Autodesk Fusion 360 part; units mm, degrees
note: some values were not read from the file. Set by a fixed rule: which sketch regions a step uses.
(part 19 of 59)
  spline S107 degree 5 poles (23.3609, -7.8781) (23.3596, -7.8757) (23.3571, -7.871) (23.3532, -7.8639) (23.348, -7.8544) (23.3416, -7.8426) (23.3351, -7.8308) (23.3287, -7.819) (23.3222, -7.8073) (23.3158, -7.7957) (23.3094, -7.784) (23.3029, -7.7724) (23.2965, -7.7609) (23.29, -7.7493) (23.2836, -7.7379) (23.2771, -7.7264) (23.2707, -7.715) (23.2643, -7.7036) (23.2578, -7.6922) (23.2514, -7.6809) (23.245, -7.6697) (23.2385, -7.6584) (23.2321, -7.6472) (23.2257, -7.636) (23.2193, -7.6249) (23.2128, -7.6138) (23.2064, -7.6028) (23.2, -7.5917) (23.1936, -7.5808) (23.1872, -7.5698) (23.1807, -7.5589) (23.1743, -7.548) (23.1679, -7.5372) (23.1615, -7.5264) (23.1551, -7.5156) (23.1487, -7.5049) (23.1423, -7.4942) (23.136, -7.4836) (23.1296, -7.473) (23.1232, -7.4624) (23.1168, -7.4518) (23.1104, -7.4413) (23.1041, -7.4309) (23.0977, -7.4205) (23.0914, -7.4101) (23.085, -7.3997) (23.0786, -7.3894) (23.0723, -7.3791) (23.066, -7.3689) (23.0596, -7.3587) (23.0533, -7.3486) (23.047, -7.3384) (23.0406, -7.3284) (23.0343, -7.3183) (23.028, -7.3083) (23.0217, -7.2984) (23.0154, -7.2884) (23.0091, -7.2785) (23.0029, -7.2687) (22.9966, -7.2589) (22.9903, -7.2491) (22.984, -7.2394) (22.9778, -7.2297) (22.9715, -7.22) (22.9653, -7.2104) (22.9591, -7.2009) (22.9528, -7.1913) (22.9466, -7.1818) (22.9404, -7.1724) (22.9342, -7.163) (22.928, -7.1536) (22.9218, -7.1443) (22.9156, -7.135) (22.9095, -7.1257) (22.9033, -7.1165) (22.8971, -7.1073) (22.891, -7.0982) (22.8849, -7.0891) (22.8787, -7.0801) (22.8726, -7.0711) (22.8665, -7.0621) (22.8604, -7.0532) (22.8543, -7.0443) (22.8483, -7.0354) (22.8422, -7.0266) (22.8361, -7.0179) (22.8301, -7.0091) (22.8241, -7.0005) (22.818, -6.9918) (22.812, -6.9832) (22.806, -6.9747) (22.8, -6.9662) (22.7941, -6.9577) (22.7881, -6.9493) (22.7822, -6.9409) (22.7762, -6.9325) (22.7703, -6.9242) (22.7644, -6.916) (22.7585, -6.9078) (22.7526, -6.8996) (22.7467, -6.8914) (22.7408, -6.8834) (22.735, -6.8753) (22.7292, -6.8673) (22.7233, -6.8593) (22.7175, -6.8514) (22.7118, -6.8436) (22.706, -6.8357) (22.7002, -6.8279) (22.6945, -6.8202) (22.6887, -6.8125) (22.683, -6.8048) (22.6773, -6.7972) (22.6716, -6.7897) (22.666, -6.7821) (22.6603, -6.7747) (22.6547, -6.7672) (22.6491, -6.7598) (22.6435, -6.7525) (22.6379, -6.7452) (22.6323, -6.7379) (22.6268, -6.7307) (22.6212, -6.7236) (22.6157, -6.7165) (22.6102, -6.7094) (22.6048, -6.7024) (22.5993, -6.6954) (22.5939, -6.6884) (22.5884, -6.6815) (22.583, -6.6747) (22.5777, -6.6679) (22.5723, -6.6611) (22.567, -6.6544) (22.5617, -6.6478) (22.5564, -6.6412) (22.5511, -6.6346) (22.5458, -6.6281) (22.5406, -6.6216) (22.5354, -6.6152) (22.5302, -6.6088) (22.525, -6.6025) (22.5199, -6.5962) (22.5148, -6.59) (22.5097, -6.5838) (22.5046, -6.5776) (22.4996, -6.5715) (22.4945, -6.5655) (22.4895, -6.5595) (22.4846, -6.5536) (22.4796, -6.5477) (22.4747, -6.5418) (22.4698, -6.536) (22.4649, -6.5303) (22.4601, -6.5246) (22.4553, -6.5189) (22.4505, -6.5133) (22.4457, -6.5077) (22.441, -6.5022) (22.4363, -6.4968) (22.4316, -6.4914) (22.427, -6.486) (22.4223, -6.4807) (22.4177, -6.4755) (22.4132, -6.4703) (22.4087, -6.4651) (22.4042, -6.46) (22.3997, -6.455) (22.3953, -6.45) (22.3909, -6.4451) (22.3865, -6.4402) (22.3821, -6.4353) (22.3778, -6.4306) (22.3736, -6.4258) (22.3693, -6.4211) (22.3651, -6.4165) (22.3609, -6.4119) (22.3568, -6.4074) (22.3527, -6.403) (22.3486, -6.3986) (22.3446, -6.3942) (22.3406, -6.3899) (22.3367, -6.3856) (22.3328, -6.3814) (22.3289, -6.3773) (22.325, -6.3732) (22.3212, -6.3692) (22.3175, -6.3652) (22.3138, -6.3613) (22.3101, -6.3574) (22.3065, -6.3536) (22.3029, -6.3499) (22.2993, -6.3462) (22.2958, -6.3426) (22.2923, -6.339) (22.2889, -6.3355) (22.2855, -6.332) (22.2822, -6.3286) (22.2789, -6.3252) (22.2757, -6.322) (22.2725, -6.3187) (22.2693, -6.3156) (22.2662, -6.3124) (22.2632, -6.3094) (22.2602, -6.3064) (22.2572, -6.3035) (22.2543, -6.3006) (22.2515, -6.2978) (22.2487, -6.2951) (22.2459, -6.2924) (22.2433, -6.2897) (22.2406, -6.2872) (22.238, -6.2847) (22.2355, -6.2823) (22.2331, -6.2799) (22.2307, -6.2776) (22.2283, -6.2753) (22.226, -6.2732) (22.2238, -6.271) (22.2216, -6.269) (22.2195, -6.267) (22.2175, -6.2651) (22.2155, -6.2632) (22.2136, -6.2615) (22.2117, -6.2597) (22.2099, -6.2581) (22.2082, -6.2565) (22.2066, -6.255) (22.205, -6.2536) (22.2035, -6.2522) (22.202, -6.2509) (22.2007, -6.2497) (22.1994, -6.2485) (22.1982, -6.2474) (22.197, -6.2464) (22.196, -6.2455) (22.195, -6.2446) (22.1941, -6.2438) (22.1933, -6.2431) (22.1925, -6.2424) (22.1919, -6.2419) (22.1913, -6.2414) (22.1909, -6.241) (22.1907, -6.2408) (22.1905, -6.2407) (22.1904, -6.2406) knots -1 -1 -1 -1 -1 -1 -0.99583333 -0.99166667 -0.9875 -0.98333333 -0.97916667 -0.975 -0.97083333 -0.96666667 -0.9625 -0.95833333 -0.95416667 -0.95 -0.94583333 -0.94166667 -0.9375 -0.93333333 -0.92916667 -0.925 -0.92083333 -0.91666667 -0.9125 -0.90833333 -0.90416667 -0.9 -0.89583333 -0.89166667 -0.8875 -0.88333333 -0.87916667 -0.875 -0.87083333 -0.86666667 -0.8625 -0.85833333 -0.85416667 -0.85 -0.84583333 -0.84166667 -0.8375 -0.83333333 -0.82916667 -0.825 -0.82083333 -0.81666667 -0.8125 -0.80833333 -0.80416667 -0.8 -0.79583333 -0.79166667 -0.7875 -0.78333333 -0.77916667 -0.775 -0.77083333 -0.76666667 -0.7625 -0.75833333 -0.75416667 -0.75 -0.74583333 -0.74166667 -0.7375 -0.73333333 -0.72916667 -0.725 -0.72083333 -0.71666667 -0.7125 -0.70833333 -0.70416667 -0.7 -0.69583333 -0.69166667 -0.6875 -0.68333333 -0.67916667 -0.675 -0.67083333 -0.66666667 -0.6625 -0.65833333 -0.65416667 -0.65 -0.64583333 -0.64166667 -0.6375 -0.63333333 -0.62916667 -0.625 -0.62083333 -0.61666667 -0.6125 -0.60833333 -0.60416667 -0.6 -0.59583333 -0.59166667 -0.5875 -0.58333333 -0.57916667 -0.575 -0.57083333 -0.56666667 -0.5625 -0.55833333 -0.55416667 -0.55 -0.54583333 -0.54166667 -0.5375 -0.53333333 -0.52916667 -0.525 -0.52083333 -0.51666667 -0.5125 -0.50833333 -0.50416667 -0.5 -0.49583333 -0.49166667 -0.4875 -0.48333333 -0.47916667 -0.475 -0.47083333 -0.46666667 -0.4625 -0.45833333 -0.45416667 -0.45 -0.44583333 -0.44166667 -0.4375 -0.43333333 -0.42916667 -0.425 -0.42083333 -0.41666667 -0.4125 -0.40833333 -0.40416667 -0.4 -0.39583333 -0.39166667 -0.3875 -0.38333333 -0.37916667 -0.375 -0.37083333 -0.36666667 -0.3625 -0.35833333 -0.35416667 -0.35 -0.34583333 -0.34166667 -0.3375 -0.33333333 -0.32916667 -0.325 -0.32083333 -0.31666667 -0.3125 -0.30833333 -0.30416667 -0.3 -0.29583333 -0.29166667 -0.2875 -0.28333333 -0.27916667 -0.275 -0.27083333 -0.26666667 -0.2625 -0.25833333 -0.25416667 -0.25 -0.24583333 -0.24166667 -0.2375 -0.23333333 -0.22916667 -0.225 -0.22083333 -0.21666667 -0.2125 -0.20833333 -0.20416667 -0.2 -0.19583333 -0.19166667 -0.1875 -0.18333333 -0.17916667 -0.175 -0.17083333 -0.16666667 -0.1625 -0.15833333 -0.15416667 -0.15 -0.14583333 -0.14166667 -0.1375 -0.13333333 -0.12916667 -0.125 -0.12083333 -0.11666667 -0.1125 -0.10833333 -0.10416667 -0.1 -0.09583333 -0.09166667 -0.0875 -0.08333333 -0.07916667 -0.075 -0.07083333 -0.06666667 -0.0625 -0.05833333 -0.05416667 -0.05 -0.04583333 -0.04166667 -0.0375 -0.03333333 -0.02916667 -0.025 -0.02083333 -0.01666667 -0.0125 -0.00833333 -0.00416667 0 0 0 0 0 0
  spline S108 degree 5 poles (-30.2174, 5.5786) (-30.2148, 5.5782) (-30.2094, 5.5775) (-30.2014, 5.5764) (-30.1907, 5.575) (-30.1773, 5.5733) (-30.164, 5.5716) (-30.1507, 5.5699) (-30.1375, 5.5683) (-30.1242, 5.5666) (-30.111, 5.565) (-30.0979, 5.5634) (-30.0847, 5.5618) (-30.0716, 5.5602) (-30.0585, 5.5587) (-30.0455, 5.5572) (-30.0324, 5.5557) (-30.0194, 5.5542) (-30.0065, 5.5527) (-29.9935, 5.5513) (-29.9806, 5.5499) (-29.9678, 5.5484) (-29.9549, 5.5471) (-29.9421, 5.5457) (-29.9293, 5.5444) (-29.9166, 5.543) (-29.9039, 5.5417) (-29.8912, 5.5404) (-29.8785, 5.5392) (-29.8659, 5.5379) (-29.8533, 5.5367) (-29.8407, 5.5355) (-29.8282, 5.5343) (-29.8157, 5.5331) (-29.8032, 5.532) (-29.7908, 5.5309) (-29.7784, 5.5298) (-29.766, 5.5287) (-29.7537, 5.5276) (-29.7414, 5.5265) (-29.7291, 5.5255) (-29.7169, 5.5245) (-29.7047, 5.5235) (-29.6925, 5.5225) (-29.6803, 5.5216) (-29.6682, 5.5206) (-29.6562, 5.5197) (-29.6441, 5.5188) (-29.6321, 5.5179) (-29.6201, 5.517) (-29.6082, 5.5162) (-29.5963, 5.5154) (-29.5844, 5.5145) (-29.5726, 5.5137) (-29.5608, 5.513) (-29.549, 5.5122) (-29.5373, 5.5115) (-29.5256, 5.5108) (-29.514, 5.51) (-29.5023, 5.5094) (-29.4907, 5.5087) (-29.4792, 5.508) (-29.4677, 5.5074) (-29.4562, 5.5068) (-29.4447, 5.5062) (-29.4333, 5.5056) (-29.422, 5.505) (-29.4106, 5.5045) (-29.3993, 5.504) (-29.3881, 5.5035) (-29.3768, 5.503) (-29.3657, 5.5025) (-29.3545, 5.502) (-29.3434, 5.5016) (-29.3323, 5.5011) (-29.3213, 5.5007) (-29.3103, 5.5003) (-29.2993, 5.4999) (-29.2884, 5.4996) (-29.2775, 5.4992) (-29.2667, 5.4989) (-29.2559, 5.4986) (-29.2451, 5.4983) (-29.2344, 5.498) (-29.2237, 5.4977) (-29.213, 5.4975) (-29.2024, 5.4972) (-29.1919, 5.497) (-29.1813, 5.4968) (-29.1708, 5.4966) (-29.1604, 5.4965) (-29.15, 5.4963) (-29.1396, 5.4962) (-29.1293, 5.496) (-29.119, 5.4959) (-29.1088, 5.4958) (-29.0986, 5.4957) (-29.0884, 5.4957) (-29.0783, 5.4956) (-29.0682, 5.4956) (-29.0582, 5.4955) (-29.0482, 5.4955) (-29.0383, 5.4955) (-29.0284, 5.4955) (-29.0185, 5.4956) (-29.0087, 5.4956) (-28.9989, 5.4957) (-28.9892, 5.4957) (-28.9795, 5.4958) (-28.9698, 5.4959) (-28.9602, 5.496) (-28.9507, 5.4962) (-28.9412, 5.4963) (-28.9317, 5.4964) (-28.9223, 5.4966) (-28.9129, 5.4968) (-28.9036, 5.497) (-28.8943, 5.4972) (-28.8851, 5.4974) (-28.8759, 5.4976) (-28.8668, 5.4979) (-28.8577, 5.4981) (-28.8486, 5.4984) (-28.8396, 5.4986) (-28.8307, 5.4989) (-28.8218, 5.4992) (-28.8129, 5.4995) (-28.8041, 5.4999) (-28.7953, 5.5002) (-28.7866, 5.5005) (-28.778, 5.5009) (-28.7694, 5.5013) (-28.7608, 5.5016) (-28.7523, 5.502) (-28.7438, 5.5024) (-28.7354, 5.5028) (-28.727, 5.5032) (-28.7187, 5.5037) (-28.7105, 5.5041) (-28.7023, 5.5046) (-28.6941, 5.505) (-28.686, 5.5055) (-28.678, 5.506) (-28.67, 5.5064) (-28.662, 5.5069) (-28.6541, 5.5074) (-28.6463, 5.5079) (-28.6385, 5.5085) (-28.6307, 5.509) (-28.6231, 5.5095) (-28.6154, 5.5101) (-28.6079, 5.5106) (-28.6004, 5.5112) (-28.5929, 5.5118) (-28.5855, 5.5123) (-28.5781, 5.5129) (-28.5709, 5.5135) (-28.5636, 5.5141) (-28.5564, 5.5147) (-28.5493, 5.5153) (-28.5423, 5.5159) (-28.5353, 5.5165) (-28.5283, 5.5172) (-28.5214, 5.5178) (-28.5146, 5.5184) (-28.5078, 5.5191) (-28.5011, 5.5197) (-28.4945, 5.5204) (-28.4879, 5.5211) (-28.4814, 5.5217) (-28.4749, 5.5224) (-28.4685, 5.5231) (-28.4622, 5.5237) (-28.4559, 5.5244) (-28.4497, 5.5251) (-28.4435, 5.5258) (-28.4374, 5.5265) (-28.4314, 5.5272) (-28.4255, 5.5279) (-28.4196, 5.5286) (-28.4137, 5.5293) (-28.408, 5.53) (-28.4023, 5.5307) (-28.3966, 5.5314) (-28.3911, 5.5321) (-28.3856, 5.5328) (-28.3802, 5.5335) (-28.3748, 5.5342) (-28.3695, 5.5349) (-28.3643, 5.5356) (-28.3592, 5.5363) (-28.3541, 5.537) (-28.3491, 5.5377) (-28.3442, 5.5384) (-28.3393, 5.5391) (-28.3345, 5.5398) (-28.3298, 5.5405) (-28.3252, 5.5412) (-28.3206, 5.5419) (-28.3161, 5.5426) (-28.3117, 5.5432) (-28.3074, 5.5439) (-28.3031, 5.5446) (-28.2989, 5.5453) (-28.2948, 5.5459) (-28.2908, 5.5466) (-28.2868, 5.5472) (-28.283, 5.5479) (-28.2792, 5.5485) (-28.2755, 5.5492) (-28.2719, 5.5498) (-28.2683, 5.5504) (-28.2649, 5.551) (-28.2615, 5.5516) (-28.2582, 5.5522) (-28.255, 5.5528) (-28.2519, 5.5534) (-28.2489, 5.5539) (-28.246, 5.5545) (-28.2431, 5.555) (-28.2404, 5.5555) (-28.2377, 5.5561) (-28.2351, 5.5566) (-28.2327, 5.5571) (-28.2303, 5.5575) (-28.228, 5.558) (-28.2258, 5.5584) (-28.2237, 5.5589) (-28.2217, 5.5593) (-28.2198, 5.5597) (-28.218, 5.5601) (-28.2163, 5.5604) (-28.2147, 5.5608) (-28.2132, 5.5611) (-28.2118, 5.5614) (-28.2106, 5.5617) (-28.2094, 5.5619) (-28.2083, 5.5622) (-28.2074, 5.5624) (-28.2065, 5.5626) (-28.2058, 5.5628) (-28.2053, 5.5629) (-28.205, 5.563) (-28.2048, 5.563) (-28.2047, 5.563) knots -1 -1 -1 -1 -1 -1 -0.99583333 -0.99166667 -0.9875 -0.98333333 -0.97916667 -0.975 -0.97083333 -0.96666667 -0.9625 -0.95833333 -0.95416667 -0.95 -0.94583333 -0.94166667 -0.9375 -0.93333333 -0.92916667 -0.925 -0.92083333 -0.91666667 -0.9125 -0.90833333 -0.90416667 -0.9 -0.89583333 -0.89166667 -0.8875 -0.88333333 -0.87916667 -0.875 -0.87083333 -0.86666667 -0.8625 -0.85833333 -0.85416667 -0.85 -0.84583333 -0.84166667 -0.8375 -0.83333333 -0.82916667 -0.825 -0.82083333 -0.81666667 -0.8125 -0.80833333 -0.80416667 -0.8 -0.79583333 -0.79166667 -0.7875 -0.78333333 -0.77916667 -0.775 -0.77083333 -0.76666667 -0.7625 -0.75833333 -0.75416667 -0.75 -0.74583333 -0.74166667 -0.7375 -0.73333333 -0.72916667 -0.725 -0.72083333 -0.71666667 -0.7125 -0.70833333 -0.70416667 -0.7 -0.69583333 -0.69166667 -0.6875 -0.68333333 -0.67916667 -0.675 -0.67083333 -0.66666667 -0.6625 -0.65833333 -0.65416667 -0.65 -0.64583333 -0.64166667 -0.6375 -0.63333333 -0.62916667 -0.625 -0.62083333 -0.61666667 -0.6125 -0.60833333 -0.60416667 -0.6 -0.59583333 -0.59166667 -0.5875 -0.58333333 -0.57916667 -0.575 -0.57083333 -0.56666667 -0.5625 -0.55833333 -0.55416667 -0.55 -0.54583333 -0.54166667 -0.5375 -0.53333333 -0.52916667 -0.525 -0.52083333 -0.51666667 -0.5125 -0.50833333 -0.50416667 -0.5 -0.49583333 -0.49166667 -0.4875 -0.48333333 -0.47916667 -0.475 -0.47083333 -0.46666667 -0.4625 -0.45833333 -0.45416667 -0.45 -0.44583333 -0.44166667 -0.4375 -0.43333333 -0.42916667 -0.425 -0.42083333 -0.41666667 -0.4125 -0.40833333 -0.40416667 -0.4 -0.39583333 -0.39166667 -0.3875 -0.38333333 -0.37916667 -0.375 -0.37083333 -0.36666667 -0.3625 -0.35833333 -0.35416667 -0.35 -0.34583333 -0.34166667 -0.3375 -0.33333333 -0.32916667 -0.325 -0.32083333 -0.31666667 -0.3125 -0.30833333 -0.30416667 -0.3 -0.29583333 -0.29166667 -0.2875 -0.28333333 -0.27916667 -0.275 -0.27083333 -0.26666667 -0.2625 -0.25833333 -0.25416667 -0.25 -0.24583333 -0.24166667 -0.2375 -0.23333333 -0.22916667 -0.225 -0.22083333 -0.21666667 -0.2125 -0.20833333 -0.20416667 -0.2 -0.19583333 -0.19166667 -0.1875 -0.18333333 -0.17916667 -0.175 -0.17083333 -0.16666667 -0.1625 -0.15833333 -0.15416667 -0.15 -0.14583333 -0.14166667 -0.1375 -0.13333333 -0.12916667 -0.125 -0.12083333 -0.11666667 -0.1125 -0.10833333 -0.10416667 -0.1 -0.09583333 -0.09166667 -0.0875 -0.08333333 -0.07916667 -0.075 -0.07083333 -0.06666667 -0.0625 -0.05833333 -0.05416667 -0.05 -0.04583333 -0.04166667 -0.0375 -0.03333333 -0.02916667 -0.025 -0.02083333 -0.01666667 -0.0125 -0.00833333 -0.00416667 0 0 0 0 0 0
  line L236 (-26.8948, 1.5341) -> (-26.8955, 1.5338)
  spline S109 degree 5 poles (18.6136, -12.2898) (18.6128, -12.2872) (18.6113, -12.282) (18.609, -12.2743) (18.6059, -12.2639) (18.6021, -12.251) (18.5982, -12.2382) (18.5943, -12.2253) (18.5905, -12.2125) (18.5866, -12.1998) (18.5827, -12.1871) (18.5788, -12.1744) (18.5749, -12.1617) (18.571, -12.1491) (18.5671, -12.1365) (18.5632, -12.124) (18.5593, -12.1115) (18.5553, -12.099) (18.5514, -12.0866) (18.5475, -12.0742) (18.5435, -12.0618) (18.5395, -12.0495) (18.5356, -12.0372) (18.5316, -12.0249) (18.5277, -12.0127) (18.5237, -12.0005) (18.5197, -11.9884) (18.5157, -11.9762) (18.5117, -11.9642) (18.5077, -11.9521) (18.5037, -11.9401) (18.4997, -11.9281) (18.4957, -11.9162) (18.4917, -11.9043) (18.4877, -11.8925) (18.4836, -11.8806) (18.4796, -11.8689) (18.4756, -11.8571) (18.4715, -11.8454) (18.4675, -11.8337) (18.4634, -11.8221) (18.4594, -11.8105) (18.4553, -11.799) (18.4513, -11.7874) (18.4472, -11.776) (18.4431, -11.7645) (18.4391, -11.7531) (18.435, -11.7417) (18.4309, -11.7304) (18.4269, -11.7191) (18.4228, -11.7079) (18.4187, -11.6967) (18.4146, -11.6855) (18.4105, -11.6744) (18.4064, -11.6633) (18.4023, -11.6522) (18.3982, -11.6412) (18.3941, -11.6302) (18.39, -11.6193) (18.3859, -11.6084) (18.3818, -11.5975) (18.3777, -11.5867) (18.3736, -11.5759) (18.3695, -11.5652) (18.3654, -11.5545) (18.3613, -11.5438) (18.3572, -11.5332) (18.3531, -11.5226) (18.349, -11.5121) (18.3449, -11.5016) (18.3408, -11.4911) (18.3366, -11.4807) (18.3325, -11.4703) (18.3284, -11.46) (18.3243, -11.4497) (18.3202, -11.4395) (18.3161, -11.4292) (18.312, -11.4191) (18.3079, -11.409) (18.3038, -11.3989) (18.2996, -11.3888) (18.2955, -11.3788) (18.2914, -11.3689) (18.2873, -11.359) (18.2832, -11.3491) (18.2791, -11.3393) (18.275, -11.3295) (18.2709, -11.3197) (18.2668, -11.31) (18.2627, -11.3004) (18.2587, -11.2907) (18.2546, -11.2812) (18.2505, -11.2716) (18.2464, -11.2622) (18.2423, -11.2527) (18.2383, -11.2433) (18.2342, -11.234) (18.2301, -11.2247) (18.226, -11.2154) (18.222, -11.2062) (18.2179, -11.197) (18.2139, -11.1879) (18.2098, -11.1788) (18.2058, -11.1697) (18.2018, -11.1607) (18.1977, -11.1518) (18.1937, -11.1429) (18.1897, -11.134) (18.1857, -11.1252) (18.1816, -11.1165) (18.1776, -11.1077) (18.1736, -11.0991) (18.1696, -11.0904) (18.1657, -11.0818) (18.1617, -11.0733) (18.1577, -11.0648) (18.1537, -11.0564) (18.1498, -11.048) (18.1458, -11.0396) (18.1419, -11.0313) (18.1379, -11.0231) (18.134, -11.0149) (18.1301, -11.0067) (18.1262, -10.9986) (18.1223, -10.9905) (18.1184, -10.9825) (18.1145, -10.9746) (18.1106, -10.9666) (18.1068, -10.9588) (18.1029, -10.951) (18.0991, -10.9432) (18.0952, -10.9355) (18.0914, -10.9278) (18.0876, -10.9202) (18.0838, -10.9126) (18.08, -10.9051) (18.0762, -10.8976) (18.0724, -10.8902) (18.0687, -10.8828) (18.0649, -10.8755) (18.0612, -10.8683) (18.0575, -10.861) (18.0538, -10.8539) (18.0501, -10.8468) (18.0464, -10.8397) (18.0427, -10.8327) (18.039, -10.8257) (18.0354, -10.8188) (18.0318, -10.812) (18.0282, -10.8052) (18.0246, -10.7984) (18.021, -10.7918) (18.0174, -10.7851) (18.0139, -10.7785) (18.0103, -10.772) (18.0068, -10.7655) (18.0033, -10.7591) (17.9998, -10.7527) (17.9963, -10.7464) (17.9929, -10.7402) (17.9895, -10.734) (17.986, -10.7278) (17.9826, -10.7217) (17.9793, -10.7157) (17.9759, -10.7097) (17.9726, -10.7038) (17.9692, -10.6979) (17.9659, -10.6921) (17.9627, -10.6864) (17.9594, -10.6807) (17.9562, -10.6751) (17.9529, -10.6695) (17.9497, -10.664) (17.9466, -10.6585) (17.9434, -10.6531) (17.9403, -10.6478) (17.9372, -10.6425) (17.9341, -10.6373) (17.931, -10.6321) (17.928, -10.627) (17.925, -10.622) (17.922, -10.617) (17.9191, -10.6121) (17.9161, -10.6072) (17.9132, -10.6024) (17.9103, -10.5977) (17.9075, -10.593) (17.9047, -10.5884) (17.9019, -10.5839) (17.8991, -10.5794) (17.8964, -10.575) (17.8937, -10.5706) (17.891, -10.5664) (17.8883, -10.5621) (17.8857, -10.558) (17.8831, -10.5539) (17.8806, -10.5499) (17.8781, -10.5459) (17.8756, -10.542) (17.8731, -10.5382) (17.8707, -10.5344) (17.8683, -10.5308) (17.866, -10.5271) (17.8637, -10.5236) (17.8614, -10.5201) (17.8592, -10.5167) (17.857, -10.5134) (17.8548, -10.5101) (17.8527, -10.5069) (17.8506, -10.5038) (17.8485, -10.5007) (17.8465, -10.4978) (17.8446, -10.4948) (17.8427, -10.492) (17.8408, -10.4893) (17.8389, -10.4866) (17.8372, -10.484) (17.8354, -10.4814) (17.8337, -10.479) (17.8321, -10.4766) (17.8305, -10.4743) (17.8289, -10.4721) (17.8274, -10.4699) (17.826, -10.4679) (17.8246, -10.4659) (17.8232, -10.464) (17.8219, -10.4622) (17.8207, -10.4604) (17.8195, -10.4588) (17.8183, -10.4572) (17.8172, -10.4557) (17.8162, -10.4543) (17.8153, -10.453) (17.8144, -10.4518) (17.8135, -10.4506) (17.8127, -10.4496) (17.812, -10.4486) (17.8114, -10.4477) (17.8108, -10.4469) (17.8103, -10.4463) (17.8098, -10.4457) (17.8095, -10.4453) (17.8093, -10.445) (17.8092, -10.4448) (17.8091, -10.4448) knots -1 -1 -1 -1 -1 -1 -0.99583333 -0.99166667 -0.9875 -0.98333333 -0.97916667 -0.975 -0.97083333 -0.96666667 -0.9625 -0.95833333 -0.95416667 -0.95 -0.94583333 -0.94166667 -0.9375 -0.93333333 -0.92916667 -0.925 -0.92083333 -0.91666667 -0.9125 -0.90833333 -0.90416667 -0.9 -0.89583333 -0.89166667 -0.8875 -0.88333333 -0.87916667 -0.875 -0.87083333 -0.86666667 -0.8625 -0.85833333 -0.85416667 -0.85 -0.84583333 -0.84166667 -0.8375 -0.83333333 -0.82916667 -0.825 -0.82083333 -0.81666667 -0.8125 -0.80833333 -0.80416667 -0.8 -0.79583333 -0.79166667 -0.7875 -0.78333333 -0.77916667 -0.775 -0.77083333 -0.76666667 -0.7625 -0.75833333 -0.75416667 -0.75 -0.74583333 -0.74166667 -0.7375 -0.73333333 -0.72916667 -0.725 -0.72083333 -0.71666667 -0.7125 -0.70833333 -0.70416667 -0.7 -0.69583333 -0.69166667 -0.6875 -0.68333333 -0.67916667 -0.675 -0.67083333 -0.66666667 -0.6625 -0.65833333 -0.65416667 -0.65 -0.64583333 -0.64166667 -0.6375 -0.63333333 -0.62916667 -0.625 -0.62083333 -0.61666667 -0.6125 -0.60833333 -0.60416667 -0.6 -0.59583333 -0.59166667 -0.5875 -0.58333333 -0.57916667 -0.575 -0.57083333 -0.56666667 -0.5625 -0.55833333 -0.55416667 -0.55 -0.54583333 -0.54166667 -0.5375 -0.53333333 -0.52916667 -0.525 -0.52083333 -0.51666667 -0.5125 -0.50833333 -0.50416667 -0.5 -0.49583333 -0.49166667 -0.4875 -0.48333333 -0.47916667 -0.475 -0.47083333 -0.46666667 -0.4625 -0.45833333 -0.45416667 -0.45 -0.44583333 -0.44166667 -0.4375 -0.43333333 -0.42916667 -0.425 -0.42083333 -0.41666667 -0.4125 -0.40833333 -0.40416667 -0.4 -0.39583333 -0.39166667 -0.3875 -0.38333333 -0.37916667 -0.375 -0.37083333 -0.36666667 -0.3625 -0.35833333 -0.35416667 -0.35 -0.34583333 -0.34166667 -0.3375 -0.33333333 -0.32916667 -0.325 -0.32083333 -0.31666667 -0.3125 -0.30833333 -0.30416667 -0.3 -0.29583333 -0.29166667 -0.2875 -0.28333333 -0.27916667 -0.275 -0.27083333 -0.26666667 -0.2625 -0.25833333 -0.25416667 -0.25 -0.24583333 -0.24166667 -0.2375 -0.23333333 -0.22916667 -0.225 -0.22083333 -0.21666667 -0.2125 -0.20833333 -0.20416667 -0.2 -0.19583333 -0.19166667 -0.1875 -0.18333333 -0.17916667 -0.175 -0.17083333 -0.16666667 -0.1625 -0.15833333 -0.15416667 -0.15 -0.14583333 -0.14166667 -0.1375 -0.13333333 -0.12916667 -0.125 -0.12083333 -0.11666667 -0.1125 -0.10833333 -0.10416667 -0.1 -0.09583333 -0.09166667 -0.0875 -0.08333333 -0.07916667 -0.075 -0.07083333 -0.06666667 -0.0625 -0.05833333 -0.05416667 -0.05 -0.04583333 -0.04166667 -0.0375 -0.03333333 -0.02916667 -0.025 -0.02083333 -0.01666667 -0.0125 -0.00833333 -0.00416667 0 0 0 0 0 0
  line L237 (-27.3243, 2.6531) -> (-27.0473, 2.7529)
  spline S110 degree 5 poles (-9.8472, -14.8251) (-9.8472, -14.8252) (-9.8473, -14.8254) (-9.8474, -14.8257) (-9.8475, -14.8262) (-9.8478, -14.8269) (-9.8481, -14.8277) (-9.8484, -14.8286) (-9.8487, -14.8296) (-9.8491, -14.8308) (-9.8495, -14.832) (-9.85, -14.8334) (-9.8505, -14.8348) (-9.851, -14.8364) (-9.8515, -14.838) (-9.8521, -14.8398) (-9.8527, -14.8416) (-9.8533, -14.8435) (-9.8539, -14.8456) (-9.8546, -14.8477) (-9.8553, -14.8499) (-9.856, -14.8523) (-9.8568, -14.8547) (-9.8575, -14.8572) (-9.8583, -14.8598) (-9.8591, -14.8625) (-9.86, -14.8652) (-9.8608, -14.8681) (-9.8617, -14.871) (-9.8626, -14.8741) (-9.8635, -14.8772) (-9.8645, -14.8804) (-9.8654, -14.8837) (-9.8664, -14.887) (-9.8674, -14.8905) (-9.8684, -14.894) (-9.8694, -14.8976) (-9.8704, -14.9013) (-9.8715, -14.9051) (-9.8725, -14.909) (-9.8736, -14.9129) (-9.8747, -14.9169) (-9.8758, -14.921) (-9.8769, -14.9252) (-9.878, -14.9294) (-9.8792, -14.9337) (-9.8803, -14.9381) (-9.8815, -14.9426) (-9.8827, -14.9471) (-9.8838, -14.9517) (-9.885, -14.9564) (-9.8862, -14.9612) (-9.8874, -14.966) (-9.8887, -14.9709) (-9.8899, -14.9759) (-9.8911, -14.981) (-9.8924, -14.9861) (-9.8936, -14.9912) (-9.8949, -14.9965) (-9.8962, -15.0018) (-9.8974, -15.0072) (-9.8987, -15.0127) (-9.9, -15.0182) (-9.9013, -15.0238) (-9.9026, -15.0294) (-9.9039, -15.0352) (-9.9052, -15.0409) (-9.9065, -15.0468) (-9.9079, -15.0527) (-9.9092, -15.0587) (-9.9105, -15.0647) (-9.9118, -15.0709) (-9.9132, -15.077) (-9.9145, -15.0833) (-9.9158, -15.0896) (-9.9172, -15.0959) (-9.9185, -15.1023) (-9.9199, -15.1088) (-9.9212, -15.1154) (-9.9225, -15.122) (-9.9239, -15.1286) (-9.9252, -15.1353) (-9.9266, -15.1421) (-9.9279, -15.149) (-9.9293, -15.1559) (-9.9306, -15.1628) (-9.932, -15.1698) (-9.9333, -15.1769) (-9.9347, -15.1841) (-9.936, -15.1912) (-9.9374, -15.1985) (-9.9387, -15.2058) (-9.9401, -15.2132) (-9.9414, -15.2206) (-9.9428, -15.228) (-9.9441, -15.2356) (-9.9454, -15.2431) (-9.9468, -15.2508) (-9.9481, -15.2585) (-9.9494, -15.2662) (-9.9508, -15.274) (-9.9521, -15.2819) (-9.9534, -15.2898) (-9.9547, -15.2977) (-9.956, -15.3057) (-9.9573, -15.3138) (-9.9586, -15.3219) (-9.9599, -15.3301) (-9.9612, -15.3383) (-9.9625, -15.3466) (-9.9638, -15.3549) (-9.9651, -15.3633) (-9.9664, -15.3717) (-9.9676, -15.3802) (-9.9689, -15.3887) (-9.9701, -15.3973) (-9.9714, -15.4059) (-9.9726, -15.4146) (-9.9739, -15.4233) (-9.9751, -15.4321) (-9.9763, -15.4409) (-9.9776, -15.4498) (-9.9788, -15.4587) (-9.98, -15.4677) (-9.9812, -15.4767) (-9.9824, -15.4858) (-9.9836, -15.4949) (-9.9847, -15.504) (-9.9859, -15.5133) (-9.9871, -15.5225) (-9.9882, -15.5318) (-9.9894, -15.5412) (-9.9905, -15.5506) (-9.9916, -15.56) (-9.9928, -15.5695) (-9.9939, -15.579) (-9.995, -15.5886) (-9.9961, -15.5982) (-9.9972, -15.6079) (-9.9983, -15.6176) (-9.9993, -15.6274) (-10.0004, -15.6372) (-10.0014, -15.647) (-10.0025, -15.6569) (-10.0035, -15.6668) (-10.0045, -15.6768) (-10.0055, -15.6868) (-10.0065, -15.6969) (-10.0075, -15.707) (-10.0085, -15.7172) (-10.0095, -15.7274) (-10.0104, -15.7376) (-10.0114, -15.7479) (-10.0123, -15.7582) (-10.0133, -15.7686) (-10.0142, -15.779) (-10.0151, -15.7894) (-10.016, -15.7999) (-10.0169, -15.8105) (-10.0177, -15.821) (-10.0186, -15.8317) (-10.0195, -15.8423) (-10.0203, -15.853) (-10.0211, -15.8638) (-10.0219, -15.8745) (-10.0227, -15.8854) (-10.0235, -15.8962) (-10.0243, -15.9071) (-10.0251, -15.9181) (-10.0258, -15.929) (-10.0266, -15.94) (-10.0273, -15.9511) (-10.028, -15.9622) (-10.0287, -15.9733) (-10.0294, -15.9845) (-10.0301, -15.9957) (-10.0308, -16.007) (-10.0314, -16.0183) (-10.0321, -16.0296) (-10.0327, -16.041) (-10.0333, -16.0524) (-10.0339, -16.0638) (-10.0345, -16.0753) (-10.0351, -16.0868) (-10.0356, -16.0984) (-10.0362, -16.11) (-10.0367, -16.1216) (-10.0372, -16.1333) (-10.0377, -16.145) (-10.0382, -16.1567) (-10.0387, -16.1685) (-10.0392, -16.1803) (-10.0396, -16.1922) (-10.04, -16.2041) (-10.0405, -16.216) (-10.0409, -16.228) (-10.0412, -16.24) (-10.0416, -16.252) (-10.042, -16.2641) (-10.0423, -16.2762) (-10.0427, -16.2883) (-10.043, -16.3005) (-10.0433, -16.3127) (-10.0436, -16.3249) (-10.0438, -16.3372) (-10.0441, -16.3495) (-10.0443, -16.3619) (-10.0445, -16.3743) (-10.0448, -16.3867) (-10.0449, -16.3991) (-10.0451, -16.4116) (-10.0453, -16.4241) (-10.0454, -16.4367) (-10.0456, -16.4493) (-10.0457, -16.4619) (-10.0458, -16.4745) (-10.0458, -16.4872) (-10.0459, -16.5) (-10.046, -16.5127) (-10.046, -16.5255) (-10.046, -16.5383) (-10.046, -16.5512) (-10.046, -16.5641) (-10.046, -16.577) (-10.0459, -16.5899) (-10.0458, -16.6029) (-10.0458, -16.6159) (-10.0457, -16.629) (-10.0455, -16.642) (-10.0454, -16.6551) (-10.0453, -16.6683) (-10.0451, -16.6815) (-10.0449, -16.6947) (-10.0447, -16.7079) (-10.0445, -16.7212) (-10.0442, -16.7345) (-10.044, -16.7478) (-10.0437, -16.7612) (-10.0434, -16.7745) (-10.0431, -16.788) (-10.0428, -16.8014) (-10.0425, -16.8122) (-10.0423, -16.8203) (-10.0422, -16.8257) (-10.0421, -16.8284) knots 0 0 0 0 0 0 0.00416667 0.00833333 0.0125 0.01666667 0.02083333 0.025 0.02916667 0.03333333 0.0375 0.04166667 0.04583333 0.05 0.05416667 0.05833333 0.0625 0.06666667 0.07083333 0.075 0.07916667 0.08333333 0.0875 0.09166667 0.09583333 0.1 0.10416667 0.10833333 0.1125 0.11666667 0.12083333 0.125 0.12916667 0.13333333 0.1375 0.14166667 0.14583333 0.15 0.15416667 0.15833333 0.1625 0.16666667 0.17083333 0.175 0.17916667 0.18333333 0.1875 0.19166667 0.19583333 0.2 0.20416667 0.20833333 0.2125 0.21666667 0.22083333 0.225 0.22916667 0.23333333 0.2375 0.24166667 0.24583333 0.25 0.25416667 0.25833333 0.2625 0.26666667 0.27083333 0.275 0.27916667 0.28333333 0.2875 0.29166667 0.29583333 0.3 0.30416667 0.30833333 0.3125 0.31666667 0.32083333 0.325 0.32916667 0.33333333 0.3375 0.34166667 0.34583333 0.35 0.35416667 0.35833333 0.3625 0.36666667 0.37083333 0.375 0.37916667 0.38333333 0.3875 0.39166667 0.39583333 0.4 0.40416667 0.40833333 0.4125 0.41666667 0.42083333 0.425 0.42916667 0.43333333 0.4375 0.44166667 0.44583333 0.45 0.45416667 0.45833333 0.4625 0.46666667 0.47083333 0.475 0.47916667 0.48333333 0.4875 0.49166667 0.49583333 0.5 0.50416667 0.50833333 0.5125 0.51666667 0.52083333 0.525 0.52916667 0.53333333 0.5375 0.54166667 0.54583333 0.55 0.55416667 0.55833333 0.5625 0.56666667 0.57083333 0.575 0.57916667 0.58333333 0.5875 0.59166667 0.59583333 0.6 0.60416667 0.60833333 0.6125 0.61666667 0.62083333 0.625 0.62916667 0.63333333 0.6375 0.64166667 0.64583333 0.65 0.65416667 0.65833333 0.6625 0.66666667 0.67083333 0.675 0.67916667 0.68333333 0.6875 0.69166667 0.69583333 0.7 0.70416667 0.70833333 0.7125 0.71666667 0.72083333 0.725 0.72916667 0.73333333 0.7375 0.74166667 0.74583333 0.75 0.75416667 0.75833333 0.7625 0.76666667 0.77083333 0.775 0.77916667 0.78333333 0.7875 0.79166667 0.79583333 0.8 0.80416667 0.80833333 0.8125 0.81666667 0.82083333 0.825 0.82916667 0.83333333 0.8375 0.84166667 0.84583333 0.85 0.85416667 0.85833333 0.8625 0.86666667 0.87083333 0.875 0.87916667 0.88333333 0.8875 0.89166667 0.89583333 0.9 0.90416667 0.90833333 0.9125 0.91666667 0.92083333 0.925 0.92916667 0.93333333 0.9375 0.94166667 0.94583333 0.95 0.95416667 0.95833333 0.9625 0.96666667 0.97083333 0.975 0.97916667 0.98333333 0.9875 0.99166667 0.99583333 1 1 1 1 1 1
  line L238 (-17.6281, -10.2115) -> (-17.8086, -10.4441)
  line L239 (-28.7745, 16.4507) -> (-28.7753, 16.4508)
  line L240 (-28.4828, 16.4106) -> (-28.7745, 16.4507)
  spline S111 degree 5 poles (20.9575, -7.61) (20.9576, -7.61) (20.9577, -7.6102) (20.958, -7.6104) (20.9583, -7.6107) (20.9589, -7.6112) (20.9595, -7.6118) (20.9602, -7.6125) (20.961, -7.6132) (20.9619, -7.614) (20.9629, -7.6149) (20.9639, -7.6159) (20.9651, -7.6169) (20.9663, -7.618) (20.9675, -7.6192) (20.9689, -7.6204) (20.9704, -7.6217) (20.9719, -7.623) (20.9735, -7.6245) (20.9752, -7.626) (20.9769, -7.6275) (20.9787, -7.6291) (20.9806, -7.6308) (20.9826, -7.6325) (20.9847, -7.6343) (20.9868, -7.6361) (20.989, -7.638) (20.9912, -7.6399) (20.9936, -7.6419) (20.996, -7.644) (20.9984, -7.6461) (21.001, -7.6482) (21.0036, -7.6504) (21.0063, -7.6527) (21.009, -7.655) (21.0119, -7.6573) (21.0148, -7.6597) (21.0177, -7.6622) (21.0207, -7.6647) (21.0238, -7.6672) (21.027, -7.6698) (21.0302, -7.6724) (21.0335, -7.6751) (21.0368, -7.6778) (21.0403, -7.6806) (21.0437, -7.6834) (21.0473, -7.6862) (21.0509, -7.6891) (21.0546, -7.692) (21.0583, -7.695) (21.0621, -7.698) (21.066, -7.701) (21.0699, -7.7041) (21.0739, -7.7072) (21.0779, -7.7103) (21.082, -7.7135) (21.0862, -7.7167) (21.0904, -7.72) (21.0947, -7.7233) (21.099, -7.7266) (21.1034, -7.73) (21.1079, -7.7333) (21.1124, -7.7368) (21.117, -7.7402) (21.1216, -7.7437) (21.1263, -7.7472) (21.1311, -7.7508) (21.1359, -7.7544) (21.1408, -7.758) (21.1457, -7.7616) (21.1507, -7.7653) (21.1557, -7.769) (21.1608, -7.7727) (21.166, -7.7765) (21.1712, -7.7802) (21.1764, -7.7841) (21.1818, -7.7879) (21.1871, -7.7918) (21.1926, -7.7956) (21.1981, -7.7996) (21.2036, -7.8035) (21.2092, -7.8075) (21.2148, -7.8115) (21.2205, -7.8155) (21.2263, -7.8195) (21.2321, -7.8236) (21.238, -7.8277) (21.2439, -7.8318) (21.2498, -7.8359) (21.2559, -7.8401) (21.2619, -7.8442) (21.2681, -7.8484) (21.2742, -7.8527) (21.2805, -7.8569) (21.2867, -7.8612) (21.2931, -7.8655) (21.2995, -7.8698) (21.3059, -7.8741) (21.3124, -7.8784) (21.3189, -7.8828) (21.3255, -7.8872) (21.3321, -7.8916) (21.3388, -7.896) (21.3455, -7.9004) (21.3523, -7.9049) (21.3592, -7.9094) (21.3661, -7.9139) (21.373, -7.9184) (21.38, -7.9229) (21.387, -7.9274) (21.3941, -7.932) (21.4012, -7.9366) (21.4084, -7.9412) (21.4156, -7.9458) (21.4229, -7.9504) (21.4302, -7.955) (21.4376, -7.9597) (21.445, -7.9644) (21.4525, -7.969) (21.46, -7.9737) (21.4676, -7.9784) (21.4752, -7.9832) (21.4828, -7.9879) (21.4905, -7.9927) (21.4983, -7.9974) (21.5061, -8.0022) (21.5139, -8.007) (21.5218, -8.0118) (21.5297, -8.0166) (21.5377, -8.0214) (21.5458, -8.0263) (21.5538, -8.0311) (21.5619, -8.036) (21.5701, -8.0409) (21.5783, -8.0457) (21.5866, -8.0506) (21.5949, -8.0555) (21.6032, -8.0605) (21.6116, -8.0654) (21.6201, -8.0703) (21.6285, -8.0753) (21.6371, -8.0802) (21.6456, -8.0852) (21.6542, -8.0902) (21.6629, -8.0951) (21.6716, -8.1001) (21.6803, -8.1051) (21.6891, -8.1101) (21.698, -8.1152) (21.7068, -8.1202) (21.7158, -8.1252) (21.7247, -8.1303) (21.7337, -8.1353) (21.7428, -8.1404) (21.7519, -8.1454) (21.761, -8.1505) (21.7702, -8.1556) (21.7794, -8.1607) (21.7887, -8.1658) (21.798, -8.1709) (21.8073, -8.176) (21.8167, -8.1811) (21.8261, -8.1862) (21.8356, -8.1913) (21.8451, -8.1965) (21.8547, -8.2016) (21.8643, -8.2067) (21.8739, -8.2119) (21.8836, -8.217) (21.8933, -8.2222) (21.9031, -8.2274) (21.9129, -8.2325) (21.9228, -8.2377) (21.9326, -8.2429) (21.9426, -8.248) (21.9525, -8.2532) (21.9625, -8.2584) (21.9726, -8.2636) (21.9827, -8.2688) (21.9928, -8.274) (22.003, -8.2792) (22.0132, -8.2844) (22.0235, -8.2896) (22.0337, -8.2948) (22.0441, -8.3) (22.0544, -8.3052) (22.0649, -8.3105) (22.0753, -8.3157) (22.0858, -8.3209) (22.0963, -8.3261) (22.1069, -8.3313) (22.1175, -8.3366) (22.1281, -8.3418) (22.1388, -8.347) (22.1496, -8.3523) (22.1603, -8.3575) (22.1711, -8.3627) (22.182, -8.368) (22.1928, -8.3732) (22.2038, -8.3784) (22.2147, -8.3837) (22.2257, -8.3889) (22.2367, -8.3942) (22.2478, -8.3994) (22.2589, -8.4046) (22.2701, -8.4099) (22.2812, -8.4151) (22.2925, -8.4204) (22.3037, -8.4256) (22.315, -8.4308) (22.3264, -8.4361) (22.3377, -8.4413) (22.3491, -8.4466) (22.3606, -8.4518) (22.3721, -8.457) (22.3836, -8.4623) (22.3951, -8.4675) (22.4067, -8.4727) (22.4184, -8.478) (22.43, -8.4832) (22.4417, -8.4884) (22.4535, -8.4937) (22.4653, -8.4989) (22.4771, -8.5041) (22.4889, -8.5093) (22.5008, -8.5145) (22.5127, -8.5198) (22.5247, -8.525) (22.5367, -8.5302) (22.5487, -8.5354) (22.5608, -8.5406) (22.5729, -8.5458) (22.585, -8.551) (22.5972, -8.5562) (22.6094, -8.5614) (22.6217, -8.5666) (22.6339, -8.5718) (22.6462, -8.577) (22.6586, -8.5822) (22.671, -8.5873) (22.6834, -8.5925) (22.6934, -8.5967) (22.7009, -8.5998) (22.7059, -8.6018) (22.7084, -8.6029) knots 0 0 0 0 0 0 0.00416667 0.00833333 0.0125 0.01666667 0.02083333 0.025 0.02916667 0.03333333 0.0375 0.04166667 0.04583333 0.05 0.05416667 0.05833333 0.0625 0.06666667 0.07083333 0.075 0.07916667 0.08333333 0.0875 0.09166667 0.09583333 0.1 0.10416667 0.10833333 0.1125 0.11666667 0.12083333 0.125 0.12916667 0.13333333 0.1375 0.14166667 0.14583333 0.15 0.15416667 0.15833333 0.1625 0.16666667 0.17083333 0.175 0.17916667 0.18333333 0.1875 0.19166667 0.19583333 0.2 0.20416667 0.20833333 0.2125 0.21666667 0.22083333 0.225 0.22916667 0.23333333 0.2375 0.24166667 0.24583333 0.25 0.25416667 0.25833333 0.2625 0.26666667 0.27083333 0.275 0.27916667 0.28333333 0.2875 0.29166667 0.29583333 0.3 0.30416667 0.30833333 0.3125 0.31666667 0.32083333 0.325 0.32916667 0.33333333 0.3375 0.34166667 0.34583333 0.35 0.35416667 0.35833333 0.3625 0.36666667 0.37083333 0.375 0.37916667 0.38333333 0.3875 0.39166667 0.39583333 0.4 0.40416667 0.40833333 0.4125 0.41666667 0.42083333 0.425 0.42916667 0.43333333 0.4375 0.44166667 0.44583333 0.45 0.45416667 0.45833333 0.4625 0.46666667 0.47083333 0.475 0.47916667 0.48333333 0.4875 0.49166667 0.49583333 0.5 0.50416667 0.50833333 0.5125 0.51666667 0.52083333 0.525 0.52916667 0.53333333 0.5375 0.54166667 0.54583333 0.55 0.55416667 0.55833333 0.5625 0.56666667 0.57083333 0.575 0.57916667 0.58333333 0.5875 0.59166667 0.59583333 0.6 0.60416667 0.60833333 0.6125 0.61666667 0.62083333 0.625 0.62916667 0.63333333 0.6375 0.64166667 0.64583333 0.65 0.65416667 0.65833333 0.6625 0.66666667 0.67083333 0.675 0.67916667 0.68333333 0.6875 0.69166667 0.69583333 0.7 0.70416667 0.70833333 0.7125 0.71666667 0.72083333 0.725 0.72916667 0.73333333 0.7375 0.74166667 0.74583333 0.75 0.75416667 0.75833333 0.7625 0.76666667 0.77083333 0.775 0.77916667 0.78333333 0.7875 0.79166667 0.79583333 0.8 0.80416667 0.80833333 0.8125 0.81666667 0.82083333 0.825 0.82916667 0.83333333 0.8375 0.84166667 0.84583333 0.85 0.85416667 0.85833333 0.8625 0.86666667 0.87083333 0.875 0.87916667 0.88333333 0.8875 0.89166667 0.89583333 0.9 0.90416667 0.90833333 0.9125 0.91666667 0.92083333 0.925 0.92916667 0.93333333 0.9375 0.94166667 0.94583333 0.95 0.95416667 0.95833333 0.9625 0.96666667 0.97083333 0.975 0.97916667 0.98333333 0.9875 0.99166667 0.99583333 1 1 1 1 1 1
  arc A119 (9.7471, -14.5473) -> (10.8547, -14.1221) centre (0, 12.5) ccw
  spline S112 degree 5 poles (6.9214, -17.7174) (6.9218, -17.7148) (6.9225, -17.7094) (6.9236, -17.7014) (6.925, -17.6907) (6.9267, -17.6773) (6.9284, -17.664) (6.9301, -17.6507) (6.9317, -17.6375) (6.9334, -17.6242) (6.935, -17.611) (6.9366, -17.5979) (6.9382, -17.5847) (6.9398, -17.5716) (6.9413, -17.5585) (6.9428, -17.5455) (6.9443, -17.5324) (6.9458, -17.5194) (6.9473, -17.5065) (6.9487, -17.4935) (6.9501, -17.4806) (6.9516, -17.4678) (6.9529, -17.4549) (6.9543, -17.4421) (6.9556, -17.4293) (6.957, -17.4166) (6.9583, -17.4039) (6.9596, -17.3912) (6.9608, -17.3785) (6.9621, -17.3659) (6.9633, -17.3533) (6.9645, -17.3407) (6.9657, -17.3282) (6.9669, -17.3157) (6.968, -17.3032) (6.9691, -17.2908) (6.9702, -17.2784) (6.9713, -17.266) (6.9724, -17.2537) (6.9735, -17.2414) (6.9745, -17.2291) (6.9755, -17.2169) (6.9765, -17.2047) (6.9775, -17.1925) (6.9784, -17.1803) (6.9794, -17.1682) (6.9803, -17.1562) (6.9812, -17.1441) (6.9821, -17.1321) (6.983, -17.1201) (6.9838, -17.1082) (6.9846, -17.0963) (6.9855, -17.0844) (6.9863, -17.0726) (6.987, -17.0608) (6.9878, -17.049) (6.9885, -17.0373) (6.9892, -17.0256) (6.99, -17.014) (6.9906, -17.0023) (6.9913, -16.9907) (6.992, -16.9792) (6.9926, -16.9677) (6.9932, -16.9562) (6.9938, -16.9447) (6.9944, -16.9333) (6.995, -16.922) (6.9955, -16.9106) (6.996, -16.8993) (6.9965, -16.8881) (6.997, -16.8768) (6.9975, -16.8657) (6.998, -16.8545) (6.9984, -16.8434) (6.9989, -16.8323) (6.9993, -16.8213) (6.9997, -16.8103) (7.0001, -16.7993) (7.0004, -16.7884) (7.0008, -16.7775) (7.0011, -16.7667) (7.0014, -16.7559) (7.0017, -16.7451) (7.002, -16.7344) (7.0023, -16.7237) (7.0025, -16.713) (7.0028, -16.7024) (7.003, -16.6919) (7.0032, -16.6813) (7.0034, -16.6708) (7.0035, -16.6604) (7.0037, -16.65) (7.0038, -16.6396) (7.004, -16.6293) (7.0041, -16.619) (7.0042, -16.6088) (7.0043, -16.5986) (7.0043, -16.5884) (7.0044, -16.5783) (7.0044, -16.5682) (7.0045, -16.5582) (7.0045, -16.5482) (7.0045, -16.5383) (7.0045, -16.5284) (7.0044, -16.5185) (7.0044, -16.5087) (7.0043, -16.4989) (7.0043, -16.4892) (7.0042, -16.4795) (7.0041, -16.4698) (7.004, -16.4602) (7.0038, -16.4507) (7.0037, -16.4412) (7.0036, -16.4317) (7.0034, -16.4223) (7.0032, -16.4129) (7.003, -16.4036) (7.0028, -16.3943) (7.0026, -16.3851) (7.0024, -16.3759) (7.0021, -16.3668) (7.0019, -16.3577) (7.0016, -16.3486) (7.0014, -16.3396) (7.0011, -16.3307) (7.0008, -16.3218) (7.0005, -16.3129) (7.0001, -16.3041) (6.9998, -16.2953) (6.9995, -16.2866) (6.9991, -16.278) (6.9987, -16.2694) (6.9984, -16.2608) (6.998, -16.2523) (6.9976, -16.2438) (6.9972, -16.2354) (6.9968, -16.227) (6.9963, -16.2187) (6.9959, -16.2105) (6.9954, -16.2023) (6.995, -16.1941) (6.9945, -16.186) (6.994, -16.178) (6.9936, -16.17) (6.9931, -16.162) (6.9926, -16.1541) (6.9921, -16.1463) (6.9915, -16.1385) (6.991, -16.1307) (6.9905, -16.1231) (6.9899, -16.1154) (6.9894, -16.1079) (6.9888, -16.1004) (6.9882, -16.0929) (6.9877, -16.0855) (6.9871, -16.0781) (6.9865, -16.0709) (6.9859, -16.0636) (6.9853, -16.0564) (6.9847, -16.0493) (6.9841, -16.0423) (6.9835, -16.0353) (6.9828, -16.0283) (6.9822, -16.0214) (6.9816, -16.0146) (6.9809, -16.0078) (6.9803, -16.0011) (6.9796, -15.9945) (6.9789, -15.9879) (6.9783, -15.9814) (6.9776, -15.9749) (6.9769, -15.9685) (6.9763, -15.9622) (6.9756, -15.9559) (6.9749, -15.9497) (6.9742, -15.9435) (6.9735, -15.9374) (6.9728, -15.9314) (6.9721, -15.9255) (6.9714, -15.9196) (6.9707, -15.9137) (6.97, -15.908) (6.9693, -15.9023) (6.9686, -15.8966) (6.9679, -15.8911) (6.9672, -15.8856) (6.9665, -15.8802) (6.9658, -15.8748) (6.9651, -15.8695) (6.9644, -15.8643) (6.9637, -15.8592) (6.963, -15.8541) (6.9623, -15.8491) (6.9616, -15.8442) (6.9609, -15.8393) (6.9602, -15.8345) (6.9595, -15.8298) (6.9588, -15.8252) (6.9581, -15.8206) (6.9574, -15.8161) (6.9568, -15.8117) (6.9561, -15.8074) (6.9554, -15.8031) (6.9547, -15.7989) (6.9541, -15.7948) (6.9534, -15.7908) (6.9528, -15.7868) (6.9521, -15.783) (6.9515, -15.7792) (6.9508, -15.7755) (6.9502, -15.7719) (6.9496, -15.7683) (6.949, -15.7649) (6.9484, -15.7615) (6.9478, -15.7582) (6.9472, -15.755) (6.9466, -15.7519) (6.9461, -15.7489) (6.9455, -15.746) (6.945, -15.7431) (6.9445, -15.7404) (6.9439, -15.7377) (6.9434, -15.7351) (6.9429, -15.7327) (6.9425, -15.7303) (6.942, -15.728) (6.9416, -15.7258) (6.9411, -15.7237) (6.9407, -15.7217) (6.9403, -15.7198) (6.9399, -15.718) (6.9396, -15.7163) (6.9392, -15.7147) (6.9389, -15.7132) (6.9386, -15.7118) (6.9383, -15.7106) (6.9381, -15.7094) (6.9378, -15.7083) (6.9376, -15.7074) (6.9374, -15.7065) (6.9372, -15.7058) (6.9371, -15.7053) (6.937, -15.705) (6.937, -15.7048) (6.937, -15.7047) knots -1 -1 -1 -1 -1 -1 -0.99583333 -0.99166667 -0.9875 -0.98333333 -0.97916667 -0.975 -0.97083333 -0.96666667 -0.9625 -0.95833333 -0.95416667 -0.95 -0.94583333 -0.94166667 -0.9375 -0.93333333 -0.92916667 -0.925 -0.92083333 -0.91666667 -0.9125 -0.90833333 -0.90416667 -0.9 -0.89583333 -0.89166667 -0.8875 -0.88333333 -0.87916667 -0.875 -0.87083333 -0.86666667 -0.8625 -0.85833333 -0.85416667 -0.85 -0.84583333 -0.84166667 -0.8375 -0.83333333 -0.82916667 -0.825 -0.82083333 -0.81666667 -0.8125 -0.80833333 -0.80416667 -0.8 -0.79583333 -0.79166667 -0.7875 -0.78333333 -0.77916667 -0.775 -0.77083333 -0.76666667 -0.7625 -0.75833333 -0.75416667 -0.75 -0.74583333 -0.74166667 -0.7375 -0.73333333 -0.72916667 -0.725 -0.72083333 -0.71666667 -0.7125 -0.70833333 -0.70416667 -0.7 -0.69583333 -0.69166667 -0.6875 -0.68333333 -0.67916667 -0.675 -0.67083333 -0.66666667 -0.6625 -0.65833333 -0.65416667 -0.65 -0.64583333 -0.64166667 -0.6375 -0.63333333 -0.62916667 -0.625 -0.62083333 -0.61666667 -0.6125 -0.60833333 -0.60416667 -0.6 -0.59583333 -0.59166667 -0.5875 -0.58333333 -0.57916667 -0.575 -0.57083333 -0.56666667 -0.5625 -0.55833333 -0.55416667 -0.55 -0.54583333 -0.54166667 -0.5375 -0.53333333 -0.52916667 -0.525 -0.52083333 -0.51666667 -0.5125 -0.50833333 -0.50416667 -0.5 -0.49583333 -0.49166667 -0.4875 -0.48333333 -0.47916667 -0.475 -0.47083333 -0.46666667 -0.4625 -0.45833333 -0.45416667 -0.45 -0.44583333 -0.44166667 -0.4375 -0.43333333 -0.42916667 -0.425 -0.42083333 -0.41666667 -0.4125 -0.40833333 -0.40416667 -0.4 -0.39583333 -0.39166667 -0.3875 -0.38333333 -0.37916667 -0.375 -0.37083333 -0.36666667 -0.3625 -0.35833333 -0.35416667 -0.35 -0.34583333 -0.34166667 -0.3375 -0.33333333 -0.32916667 -0.325 -0.32083333 -0.31666667 -0.3125 -0.30833333 -0.30416667 -0.3 -0.29583333 -0.29166667 -0.2875 -0.28333333 -0.27916667 -0.275 -0.27083333 -0.26666667 -0.2625 -0.25833333 -0.25416667 -0.25 -0.24583333 -0.24166667 -0.2375 -0.23333333 -0.22916667 -0.225 -0.22083333 -0.21666667 -0.2125 -0.20833333 -0.20416667 -0.2 -0.19583333 -0.19166667 -0.1875 -0.18333333 -0.17916667 -0.175 -0.17083333 -0.16666667 -0.1625 -0.15833333 -0.15416667 -0.15 -0.14583333 -0.14166667 -0.1375 -0.13333333 -0.12916667 -0.125 -0.12083333 -0.11666667 -0.1125 -0.10833333 -0.10416667 -0.1 -0.09583333 -0.09166667 -0.0875 -0.08333333 -0.07916667 -0.075 -0.07083333 -0.06666667 -0.0625 -0.05833333 -0.05416667 -0.05 -0.04583333 -0.04166667 -0.0375 -0.03333333 -0.02916667 -0.025 -0.02083333 -0.01666667 -0.0125 -0.00833333 -0.00416667 0 0 0 0 0 0
  line L241 (27.8937, 4.4055) -> (27.6109, 4.4875)
  arc A120 (28.7355, 13.4119) -> (28.6734, 14.5967) centre (0, 12.5) ccw